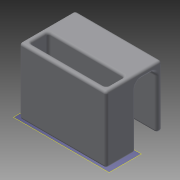
# Autodesk Inventor part: sd.adapter
Saved by Autodesk Inventor 2015 (Build 190159000, 159)
## iProperties
Created: 2016-09-03
Part Number: sd.adapter
Material: Generic
Document SubType Name: Modeling
Designer: Administrator
Density: 1 g/cm^3
Appearance: Default
Author: Administrator
Autodesk Inventor part; units mm, degrees
ref_plane "YZ Plane" through (0, 0, 0) normal (1, 0, 0) x (0, 1, 0)
ref_plane "XZ Plane" through (0, 0, 0) normal (0, 1, 0) x (-1, 0, 0)
ref_plane "XY Plane" through (0, 0, 0) normal (0, 0, 1) x (1, 0, 0)
sketch "Sketch1" plane through (0, 0, 0) normal (0, 0, 1) x (1, 0, 0)
  line L0 (-20.02, 0) -> (20.02, 0) projected
  line L1 (0, -8.48) -> (0, 17.28) projected
  line L2 (-12.5, 3) -> (12.5, 3)
  line L3 (12.5, 3) -> (12.5, -3)
  line L4 (12.5, -3) -> (-12.5, -3)
  line L5 (-12.5, -3) -> (-12.5, 3)
  line L6 (14.3, 4.8) -> (-14.3, 4.8)
  line L7 (-14.3, 4.8) -> (-14.3, -4.8)
  line L8 (-14.3, -4.8) -> (14.3, -4.8)
  line L9 (14.3, -4.8) -> (14.3, 4.8)
  point P0 (0, 0)
  dimension "d0" = 1.8
  dimension "d1" = 25
  dimension "d2" = 6
  constraints: 16 end point, 4 parallel, 2 perpendicular, 2 symmetric about line, 1 horizontal, 3 other
  measures "d0" distance between parallel lines of L2 L6
  measures "d1" distance of L2.start L2.end
  measures "d2" distance of L4.end L2.start
extrude "Extrusion1" add sketch "Sketch1" along normal blind 20 contours L7 L6 L1 L2 L5 L0 | L0 L5 L4 L1 L8 L7 | L6 L9 L0 L3 L2 L1 | L1 L4 L3 L0 L9 L8
ref_plane "Work Plane1" through (0, 0, -1.8) normal (0, 0, -1) x (-1, 0, 0)
sketch "Sketch3" plane through (0, 0, -1.8) normal (0, 0, -1) x (-1, 0, 0)
  line L0 (-14.3, -4.8) -> (-14.3, 4.8) projected
  line L1 (-12.5, -3) -> (-12.5, 3) projected
  line L2 (-12.5, 3) -> (12.5, 3) projected
  line L3 (12.5, 3) -> (12.5, -3) projected
  line L4 (12.5, -3) -> (-12.5, -3) projected
  line L5 (-14.3, 4.8) -> (14.3, 4.8) projected
  line L6 (-14.3, -4.8) -> (-14.3, 4.8) projected
  line L7 (14.3, -4.8) -> (-14.3, -4.8) projected
  line L8 (14.3, 4.8) -> (14.3, -4.8) projected
  point P0 (0, 0)
extrude "Extrusion2" add sketch "Sketch3" against normal blind 1.8 contours L0 L5 L8 L7 | L1 L2 L3 L4
sketch "Sketch2" plane through (14.3, -4.8, 0) normal (1, 0, 0) x (0, 0, -1)
  line L0 (0, 1.8) -> (-20, 1.8) projected
  line L1 (1.8, 9.6) -> (-20, 9.6) projected
  line L2 (-20, 0) -> (-20, 9.6) projected
  line L3 (1.8, 0) -> (-20, 0) projected
  line L4 (-20, 9.6) -> (-20, 18.4)
  line L5 (-20, 18.4) -> (0, 18.4)
  line L6 (0, 18.4) -> (0, 16.6)
  line L7 (0, 16.6) -> (-18.2, 16.6)
  line L8 (-18.2, 16.6) -> (-18.2, 9.6)
  line L9 (1.8, 9.6) -> (1.8, 0) projected
  point P0 (0, 4.8)
  dimension "d5" = 1.8
  dimension "d6" = 1.8
  dimension "d7" = 7
  constraints: 10 end point, 4 perpendicular, 1 point on line, 1 vertical
  measures "d5" distance of L5.end L6.end
  measures "d6" distance between parallel lines of L8 L4
  measures "d7" distance between parallel lines of L1 L7
extrude "Extrusion3" add sketch "Sketch2" against normal blind 28.6 contours L1 L4 L5 L6 L7 L8
fillet "Fillet1" radius 2 2 edges at (0, 4.8, 18.2) (0, 11.8, 18.2)
fillet "Fillet2" radius 0.8 33 edges at (14.3, 4.4, 20) (14.3, 13.6, 10) (14.3, 8.3, 18.2) (14.3, 11.8, 8.1) (14.3, 4.8, 7.2) (14.3, -4.8, 9.1) (14.3, 0, -1.8) (0, 4.8, -1.8) (-14.3, 8.3, 18.2) (-14.3, 11.8, 8.1) (-14.3, 4.8, 7.2) (0, 11.8, 0) (14.3, 12.7, 0) (0, 13.6, 0) (-14.3, 12.7, 0) (0, 13.6, 20) (-14.3, 13.6, 10) (-14.3, 4.4, 20) (0, -4.8, 20) (-14.3, -4.8, 9.1) (0, -4.8, -1.8) (-14.3, 0, -1.8) (0, -3, 20) (12.5, 0, 20) (0, 3, 20) (-12.5, 0, 20) (-12.5, -3, 10) (0, -3, 0) (-12.5, 0, 0) (-12.5, 3, 10) (0, 3, 0) (12.5, -3, 10) (12.5, 3, 10)
body "Solid1"
